Autodesk Fusion 360 part; units mm, degrees
(part 4 of 40)
  spline S18 degree 5 poles (171.8057, 195.8153) (171.7853, 195.8385) (171.7452, 195.8854) (171.6869, 195.9573) (171.6128, 196.056) (171.5254, 196.1833) (171.4416, 196.3135) (171.36, 196.4454) (171.2796, 196.5782) (171.2, 196.7117) (171.1213, 196.8458) (171.0437, 196.9807) (170.9678, 197.1168) (170.8937, 197.2543) (170.8214, 197.393) (170.7507, 197.5329) (170.6816, 197.6738) (170.6136, 197.8156) (170.5467, 197.9581) (170.4808, 198.1012) (170.416, 198.245) (170.3522, 198.3895) (170.2896, 198.5347) (170.2281, 198.6807) (170.1678, 198.8274) (170.1086, 198.9749) (170.0505, 199.123) (169.9934, 199.2717) (169.9373, 199.421) (169.8821, 199.5709) (169.8279, 199.7214) (169.7746, 199.8724) (169.7223, 200.024) (169.671, 200.1761) (169.6206, 200.3288) (169.5712, 200.482) (169.5226, 200.6358) (169.475, 200.79) (169.4283, 200.9447) (169.3825, 201.0999) (169.3375, 201.2556) (169.2934, 201.4118) (169.2502, 201.5684) (169.2079, 201.7255) (169.1664, 201.883) (169.1257, 202.0409) (169.0859, 202.1993) (169.047, 202.3581) (169.0089, 202.5173) (168.9716, 202.6769) (168.9351, 202.8369) (168.8994, 202.9973) (168.8646, 203.1581) (168.8305, 203.3193) (168.7973, 203.4809) (168.7648, 203.6428) (168.7332, 203.8051) (168.7023, 203.9677) (168.6723, 204.1307) (168.643, 204.294) (168.6145, 204.4577) (168.5867, 204.6217) (168.5597, 204.7861) (168.5336, 204.9508) (168.5081, 205.1158) (168.4834, 205.2811) (168.4595, 205.4467) (168.4364, 205.6126) (168.414, 205.7789) (168.3923, 205.9454) (168.3714, 206.1122) (168.3553, 206.2459) (168.3435, 206.3463) (168.3358, 206.4133) (168.332, 206.4469) knots 0 0 0 0 0 0 0.01428571 0.02857143 0.04285714 0.05714286 0.07142857 0.08571429 0.1 0.11428571 0.12857143 0.14285714 0.15714286 0.17142857 0.18571429 0.2 0.21428571 0.22857143 0.24285714 0.25714286 0.27142857 0.28571429 0.3 0.31428571 0.32857143 0.34285714 0.35714286 0.37142857 0.38571429 0.4 0.41428571 0.42857143 0.44285714 0.45714286 0.47142857 0.48571429 0.5 0.51428571 0.52857143 0.54285714 0.55714286 0.57142857 0.58571429 0.6 0.61428571 0.62857143 0.64285714 0.65714286 0.67142857 0.68571429 0.7 0.71428571 0.72857143 0.74285714 0.75714286 0.77142857 0.78571429 0.8 0.81428571 0.82857143 0.84285714 0.85714286 0.87142857 0.88571429 0.9 0.91428571 0.92857143 0.94285714 0.95714286 0.97142857 0.98571429 1 1 1 1 1 1
  line L1367 (171.8057, 195.8153) -> (171.7853, 195.8385) construction
  line L1368 (171.7853, 195.8385) -> (171.7452, 195.8854) construction
  line L1369 (171.7452, 195.8854) -> (171.6869, 195.9573) construction
  line L1370 (171.6869, 195.9573) -> (171.6128, 196.056) construction
  line L1371 (171.6128, 196.056) -> (171.5254, 196.1833) construction
  line L1372 (171.5254, 196.1833) -> (171.4416, 196.3135) construction
  line L1373 (171.4416, 196.3135) -> (171.36, 196.4454) construction
  line L1374 (171.36, 196.4454) -> (171.2796, 196.5782) construction
  line L1375 (171.2796, 196.5782) -> (171.2, 196.7117) construction
  line L1376 (171.2, 196.7117) -> (171.1213, 196.8458) construction
  line L1377 (171.1213, 196.8458) -> (171.0437, 196.9807) construction
  line L1378 (171.0437, 196.9807) -> (170.9678, 197.1168) construction
  line L1379 (170.9678, 197.1168) -> (170.8937, 197.2543) construction
  line L1380 (170.8937, 197.2543) -> (170.8214, 197.393) construction
  line L1381 (170.8214, 197.393) -> (170.7507, 197.5329) construction
  line L1382 (170.7507, 197.5329) -> (170.6816, 197.6738) construction
  line L1383 (170.6816, 197.6738) -> (170.6136, 197.8156) construction
  line L1384 (170.6136, 197.8156) -> (170.5467, 197.9581) construction
  line L1385 (170.5467, 197.9581) -> (170.4808, 198.1012) construction
  line L1386 (170.4808, 198.1012) -> (170.416, 198.245) construction
  line L1387 (170.416, 198.245) -> (170.3522, 198.3895) construction
  line L1388 (170.3522, 198.3895) -> (170.2896, 198.5347) construction
  line L1389 (170.2896, 198.5347) -> (170.2281, 198.6807) construction
  line L1390 (170.2281, 198.6807) -> (170.1678, 198.8274) construction
  line L1391 (170.1678, 198.8274) -> (170.1086, 198.9749) construction
  line L1392 (170.1086, 198.9749) -> (170.0505, 199.123) construction
  line L1393 (170.0505, 199.123) -> (169.9934, 199.2717) construction
  line L1394 (169.9934, 199.2717) -> (169.9373, 199.421) construction
  line L1395 (169.9373, 199.421) -> (169.8821, 199.5709) construction
  line L1396 (169.8821, 199.5709) -> (169.8279, 199.7214) construction
  line L1397 (169.8279, 199.7214) -> (169.7746, 199.8724) construction
  line L1398 (169.7746, 199.8724) -> (169.7223, 200.024) construction
  line L1399 (169.7223, 200.024) -> (169.671, 200.1761) construction
  line L1400 (169.671, 200.1761) -> (169.6206, 200.3288) construction
  line L1401 (169.6206, 200.3288) -> (169.5712, 200.482) construction
  line L1402 (169.5712, 200.482) -> (169.5226, 200.6358) construction
  line L1403 (169.5226, 200.6358) -> (169.475, 200.79) construction
  line L1404 (169.475, 200.79) -> (169.4283, 200.9447) construction
  line L1405 (169.4283, 200.9447) -> (169.3825, 201.0999) construction
  line L1406 (169.3825, 201.0999) -> (169.3375, 201.2556) construction
  line L1407 (169.3375, 201.2556) -> (169.2934, 201.4118) construction
  line L1408 (169.2934, 201.4118) -> (169.2502, 201.5684) construction
  line L1409 (169.2502, 201.5684) -> (169.2079, 201.7255) construction
  line L1410 (169.2079, 201.7255) -> (169.1664, 201.883) construction
  line L1411 (169.1664, 201.883) -> (169.1257, 202.0409) construction
  line L1412 (169.1257, 202.0409) -> (169.0859, 202.1993) construction
  line L1413 (169.0859, 202.1993) -> (169.047, 202.3581) construction
  line L1414 (169.047, 202.3581) -> (169.0089, 202.5173) construction
  line L1415 (169.0089, 202.5173) -> (168.9716, 202.6769) construction
  line L1416 (168.9716, 202.6769) -> (168.9351, 202.8369) construction
  line L1417 (168.9351, 202.8369) -> (168.8994, 202.9973) construction
  line L1418 (168.8994, 202.9973) -> (168.8646, 203.1581) construction
  line L1419 (168.8646, 203.1581) -> (168.8305, 203.3193) construction
  line L1420 (168.8305, 203.3193) -> (168.7973, 203.4809) construction
  line L1421 (168.7973, 203.4809) -> (168.7648, 203.6428) construction
  line L1422 (168.7648, 203.6428) -> (168.7332, 203.8051) construction
  line L1423 (168.7332, 203.8051) -> (168.7023, 203.9677) construction
  line L1424 (168.7023, 203.9677) -> (168.6723, 204.1307) construction
  line L1425 (168.6723, 204.1307) -> (168.643, 204.294) construction
  line L1426 (168.643, 204.294) -> (168.6145, 204.4577) construction
  line L1427 (168.6145, 204.4577) -> (168.5867, 204.6217) construction
  line L1428 (168.5867, 204.6217) -> (168.5597, 204.7861) construction
  line L1429 (168.5597, 204.7861) -> (168.5336, 204.9508) construction
  line L1430 (168.5336, 204.9508) -> (168.5081, 205.1158) construction
  line L1431 (168.5081, 205.1158) -> (168.4834, 205.2811) construction
  line L1432 (168.4834, 205.2811) -> (168.4595, 205.4467) construction
  line L1433 (168.4595, 205.4467) -> (168.4364, 205.6126) construction
  line L1434 (168.4364, 205.6126) -> (168.414, 205.7789) construction
  line L1435 (168.414, 205.7789) -> (168.3923, 205.9454) construction
  line L1436 (168.3923, 205.9454) -> (168.3714, 206.1122) construction
  line L1437 (168.3714, 206.1122) -> (168.3553, 206.2459) construction
  line L1438 (168.3553, 206.2459) -> (168.3435, 206.3463) construction
  line L1439 (168.3435, 206.3463) -> (168.3358, 206.4133) construction
  line L1440 (168.3358, 206.4133) -> (168.332, 206.4469) construction
  spline S19 degree 5 poles (171.8057, 195.8153) (171.7853, 195.8385) (171.7452, 195.8854) (171.6869, 195.9573) (171.6128, 196.056) (171.5254, 196.1833) (171.4416, 196.3135) (171.36, 196.4454) (171.2796, 196.5782) (171.2, 196.7117) (171.1213, 196.8458) (171.0437, 196.9807) (170.9678, 197.1168) (170.8937, 197.2543) (170.8214, 197.393) (170.7507, 197.5329) (170.6816, 197.6738) (170.6136, 197.8156) (170.5467, 197.9581) (170.4808, 198.1012) (170.416, 198.245) (170.3522, 198.3895) (170.2896, 198.5347) (170.2281, 198.6807) (170.1678, 198.8274) (170.1086, 198.9749) (170.0505, 199.123) (169.9934, 199.2717) (169.9373, 199.421) (169.8821, 199.5709) (169.8279, 199.7214) (169.7746, 199.8724) (169.7223, 200.024) (169.671, 200.1761) (169.6206, 200.3288) (169.5712, 200.482) (169.5226, 200.6358) (169.475, 200.79) (169.4283, 200.9447) (169.3825, 201.0999) (169.3375, 201.2556) (169.2934, 201.4118) (169.2502, 201.5684) (169.2079, 201.7255) (169.1664, 201.883) (169.1257, 202.0409) (169.0859, 202.1993) (169.047, 202.3581) (169.0089, 202.5173) (168.9716, 202.6769) (168.9351, 202.8369) (168.8994, 202.9973) (168.8646, 203.1581) (168.8305, 203.3193) (168.7973, 203.4809) (168.7648, 203.6428) (168.7332, 203.8051) (168.7023, 203.9677) (168.6723, 204.1307) (168.643, 204.294) (168.6145, 204.4577) (168.5867, 204.6217) (168.5597, 204.7861) (168.5336, 204.9508) (168.5081, 205.1158) (168.4834, 205.2811) (168.4595, 205.4467) (168.4364, 205.6126) (168.414, 205.7789) (168.3923, 205.9454) (168.3714, 206.1122) (168.3553, 206.2459) (168.3435, 206.3463) (168.3358, 206.4133) (168.332, 206.4469) knots 0 0 0 0 0 0 0.01428571 0.02857143 0.04285714 0.05714286 0.07142857 0.08571429 0.1 0.11428571 0.12857143 0.14285714 0.15714286 0.17142857 0.18571429 0.2 0.21428571 0.22857143 0.24285714 0.25714286 0.27142857 0.28571429 0.3 0.31428571 0.32857143 0.34285714 0.35714286 0.37142857 0.38571429 0.4 0.41428571 0.42857143 0.44285714 0.45714286 0.47142857 0.48571429 0.5 0.51428571 0.52857143 0.54285714 0.55714286 0.57142857 0.58571429 0.6 0.61428571 0.62857143 0.64285714 0.65714286 0.67142857 0.68571429 0.7 0.71428571 0.72857143 0.74285714 0.75714286 0.77142857 0.78571429 0.8 0.81428571 0.82857143 0.84285714 0.85714286 0.87142857 0.88571429 0.9 0.91428571 0.92857143 0.94285714 0.95714286 0.97142857 0.98571429 1 1 1 1 1 1
  line L1441 (171.8057, 195.8153) -> (171.7853, 195.8385) construction
  line L1442 (171.7853, 195.8385) -> (171.7452, 195.8854) construction
  line L1443 (171.7452, 195.8854) -> (171.6869, 195.9573) construction
  line L1444 (171.6869, 195.9573) -> (171.6128, 196.056) construction
  line L1445 (171.6128, 196.056) -> (171.5254, 196.1833) construction
  line L1446 (171.5254, 196.1833) -> (171.4416, 196.3135) construction
  line L1447 (171.4416, 196.3135) -> (171.36, 196.4454) construction
  line L1448 (171.36, 196.4454) -> (171.2796, 196.5782) construction
  line L1449 (171.2796, 196.5782) -> (171.2, 196.7117) construction
  line L1450 (171.2, 196.7117) -> (171.1213, 196.8458) construction
  line L1451 (171.1213, 196.8458) -> (171.0437, 196.9807) construction
  line L1452 (171.0437, 196.9807) -> (170.9678, 197.1168) construction
  line L1453 (170.9678, 197.1168) -> (170.8937, 197.2543) construction
  line L1454 (170.8937, 197.2543) -> (170.8214, 197.393) construction
  line L1455 (170.8214, 197.393) -> (170.7507, 197.5329) construction
  line L1456 (170.7507, 197.5329) -> (170.6816, 197.6738) construction
  line L1457 (170.6816, 197.6738) -> (170.6136, 197.8156) construction
  line L1458 (170.6136, 197.8156) -> (170.5467, 197.9581) construction
  line L1459 (170.5467, 197.9581) -> (170.4808, 198.1012) construction
  line L1460 (170.4808, 198.1012) -> (170.416, 198.245) construction
  line L1461 (170.416, 198.245) -> (170.3522, 198.3895) construction
  line L1462 (170.3522, 198.3895) -> (170.2896, 198.5347) construction
  line L1463 (170.2896, 198.5347) -> (170.2281, 198.6807) construction
  line L1464 (170.2281, 198.6807) -> (170.1678, 198.8274) construction
  line L1465 (170.1678, 198.8274) -> (170.1086, 198.9749) construction
  line L1466 (170.1086, 198.9749) -> (170.0505, 199.123) construction
  line L1467 (170.0505, 199.123) -> (169.9934, 199.2717) construction
  line L1468 (169.9934, 199.2717) -> (169.9373, 199.421) construction
  line L1469 (169.9373, 199.421) -> (169.8821, 199.5709) construction
  line L1470 (169.8821, 199.5709) -> (169.8279, 199.7214) construction
  line L1471 (169.8279, 199.7214) -> (169.7746, 199.8724) construction
  line L1472 (169.7746, 199.8724) -> (169.7223, 200.024) construction
  line L1473 (169.7223, 200.024) -> (169.671, 200.1761) construction
  line L1474 (169.671, 200.1761) -> (169.6206, 200.3288) construction
  line L1475 (169.6206, 200.3288) -> (169.5712, 200.482) construction
  line L1476 (169.5712, 200.482) -> (169.5226, 200.6358) construction
  line L1477 (169.5226, 200.6358) -> (169.475, 200.79) construction
  line L1478 (169.475, 200.79) -> (169.4283, 200.9447) construction
  line L1479 (169.4283, 200.9447) -> (169.3825, 201.0999) construction
  line L1480 (169.3825, 201.0999) -> (169.3375, 201.2556) construction
  line L1481 (169.3375, 201.2556) -> (169.2934, 201.4118) construction
  line L1482 (169.2934, 201.4118) -> (169.2502, 201.5684) construction
  line L1483 (169.2502, 201.5684) -> (169.2079, 201.7255) construction
  line L1484 (169.2079, 201.7255) -> (169.1664, 201.883) construction
  line L1485 (169.1664, 201.883) -> (169.1257, 202.0409) construction
  line L1486 (169.1257, 202.0409) -> (169.0859, 202.1993) construction
  line L1487 (169.0859, 202.1993) -> (169.047, 202.3581) construction
  line L1488 (169.047, 202.3581) -> (169.0089, 202.5173) construction
  line L1489 (169.0089, 202.5173) -> (168.9716, 202.6769) construction
  line L1490 (168.9716, 202.6769) -> (168.9351, 202.8369) construction
  line L1491 (168.9351, 202.8369) -> (168.8994, 202.9973) construction
  line L1492 (168.8994, 202.9973) -> (168.8646, 203.1581) construction
  line L1493 (168.8646, 203.1581) -> (168.8305, 203.3193) construction
  line L1494 (168.8305, 203.3193) -> (168.7973, 203.4809) construction
  line L1495 (168.7973, 203.4809) -> (168.7648, 203.6428) construction
  line L1496 (168.7648, 203.6428) -> (168.7332, 203.8051) construction
  line L1497 (168.7332, 203.8051) -> (168.7023, 203.9677) construction
  line L1498 (168.7023, 203.9677) -> (168.6723, 204.1307) construction
  line L1499 (168.6723, 204.1307) -> (168.643, 204.294) construction
  line L1500 (168.643, 204.294) -> (168.6145, 204.4577) construction
  line L1501 (168.6145, 204.4577) -> (168.5867, 204.6217) construction
  line L1502 (168.5867, 204.6217) -> (168.5597, 204.7861) construction
  line L1503 (168.5597, 204.7861) -> (168.5336, 204.9508) construction
  line L1504 (168.5336, 204.9508) -> (168.5081, 205.1158) construction
  line L1505 (168.5081, 205.1158) -> (168.4834, 205.2811) construction
  line L1506 (168.4834, 205.2811) -> (168.4595, 205.4467) construction
  line L1507 (168.4595, 205.4467) -> (168.4364, 205.6126) construction
  line L1508 (168.4364, 205.6126) -> (168.414, 205.7789) construction
  line L1509 (168.414, 205.7789) -> (168.3923, 205.9454) construction
  line L1510 (168.3923, 205.9454) -> (168.3714, 206.1122) construction
  line L1511 (168.3714, 206.1122) -> (168.3553, 206.2459) construction
  line L1512 (168.3553, 206.2459) -> (168.3435, 206.3463) construction
  line L1513 (168.3435, 206.3463) -> (168.3358, 206.4133) construction
  line L1514 (168.3358, 206.4133) -> (168.332, 206.4469) construction
  arc A49 (242.4118, 98.8934) -> (239.7302, 99.6279) centre (240.6912, 97.8739) ccw
  arc A50 (242.4118, 98.8934) -> (239.7302, 99.6279) centre (240.6912, 97.8739) ccw
  line L1515 (251.3803, 105.4094) -> (252.4583, 104.1847)
  line L1516 (251.3803, 105.4094) -> (252.4583, 104.1847)
  line L1517 (242.4118, 98.8934) -> (243.2435, 97.4897)
  line L1518 (242.4118, 98.8934) -> (243.2435, 97.4897)
  arc A51 (236.6621, 98.0646) -> (239.7302, 99.6279) centre (212.132, 150) ccw
  arc A52 (251.5104, 108.1868) -> (251.3803, 105.4094) centre (252.8816, 106.7308) ccw
  arc A53 (264.0674, 174.5301) -> (262.5041, 177.5982) centre (212.132, 150) ccw
  arc A54 (236.6621, 98.0646) -> (239.7302, 99.6279) centre (212.132, 150) ccw
  arc A55 (264.0674, 174.5301) -> (266.6686, 173.5481) centre (265.8758, 175.3842) ccw
  arc A56 (251.5104, 108.1868) -> (251.3803, 105.4094) centre (252.8816, 106.7308) ccw
  spline S20 degree 5 poles (272.9005, 144.3049) (272.9313, 144.3021) (272.9929, 144.2971) (273.0853, 144.2922) (273.2086, 144.2903) (273.363, 144.2944) (273.5176, 144.3031) (273.6723, 144.3146) (273.827, 144.3277) (273.9818, 144.3417) (274.1365, 144.3569) (274.2913, 144.3735) (274.446, 144.392) (274.6008, 144.4129) (274.7555, 144.4359) (274.9102, 144.461) (275.0649, 144.4879) (275.2195, 144.5162) (275.3741, 144.5458) (275.5286, 144.5767) (275.6831, 144.6087) (275.8375, 144.6421) (275.9918, 144.6768) (276.146, 144.7129) (276.3002, 144.7503) (276.4542, 144.7891) (276.6082, 144.8291) (276.7621, 144.8703) (276.9159, 144.9127) (277.0696, 144.9561) (277.2232, 145.0007) (277.3767, 145.0464) (277.53, 145.0932) (277.6833, 145.1411) (277.8364, 145.1901) (277.9894, 145.2401) (278.1423, 145.2913) (278.2951, 145.3434) (278.4478, 145.3965) (278.6003, 145.4507) (278.7526, 145.5058) (278.9049, 145.562) (279.057, 145.619) (279.209, 145.6771) (279.3608, 145.7361) (279.5124, 145.7961) (279.664, 145.857) (279.8153, 145.9188) (279.9665, 145.9815) (280.1176, 146.0452) (280.2685, 146.1097) (280.4192, 146.1751) (280.5698, 146.2415) (280.7202, 146.3087) (280.8704, 146.3767) (281.0205, 146.4457) (281.1704, 146.5154) (281.3201, 146.5861) (281.4696, 146.6575) (281.619, 146.7299) (281.7682, 146.803) (281.9172, 146.877) (282.066, 146.9518) (282.2146, 147.0274) (282.3631, 147.1038) (282.5113, 147.181) (282.6594, 147.259) (282.8072, 147.3378) (282.9549, 147.4174) (283.1023, 147.4977) (283.2496, 147.5789) (283.3672, 147.6444) (283.4554, 147.6939) (283.5141, 147.7271) (283.5435, 147.7437) knots 0 0 0 0 0 0 0.01428571 0.02857143 0.04285714 0.05714286 0.07142857 0.08571429 0.1 0.11428571 0.12857143 0.14285714 0.15714286 0.17142857 0.18571429 0.2 0.21428571 0.22857143 0.24285714 0.25714286 0.27142857 0.28571429 0.3 0.31428571 0.32857143 0.34285714 0.35714286 0.37142857 0.38571429 0.4 0.41428571 0.42857143 0.44285714 0.45714286 0.47142857 0.48571429 0.5 0.51428571 0.52857143 0.54285714 0.55714286 0.57142857 0.58571429 0.6 0.61428571 0.62857143 0.64285714 0.65714286 0.67142857 0.68571429 0.7 0.71428571 0.72857143 0.74285714 0.75714286 0.77142857 0.78571429 0.8 0.81428571 0.82857143 0.84285714 0.85714286 0.87142857 0.88571429 0.9 0.91428571 0.92857143 0.94285714 0.95714286 0.97142857 0.98571429 1 1 1 1 1 1
  line L1519 (272.9005, 144.3049) -> (272.9313, 144.3021) construction
  line L1520 (272.9313, 144.3021) -> (272.9929, 144.2971) construction
  line L1521 (272.9929, 144.2971) -> (273.0853, 144.2922) construction
  line L1522 (273.0853, 144.2922) -> (273.2086, 144.2903) construction
  line L1523 (273.2086, 144.2903) -> (273.363, 144.2944) construction
  line L1524 (273.363, 144.2944) -> (273.5176, 144.3031) construction
  line L1525 (273.5176, 144.3031) -> (273.6723, 144.3146) construction
  line L1526 (273.6723, 144.3146) -> (273.827, 144.3277) construction
  line L1527 (273.827, 144.3277) -> (273.9818, 144.3417) construction
  line L1528 (273.9818, 144.3417) -> (274.1365, 144.3569) construction
  line L1529 (274.1365, 144.3569) -> (274.2913, 144.3735) construction
  line L1530 (274.2913, 144.3735) -> (274.446, 144.392) construction
  line L1531 (274.446, 144.392) -> (274.6008, 144.4129) construction
  line L1532 (274.6008, 144.4129) -> (274.7555, 144.4359) construction
  line L1533 (274.7555, 144.4359) -> (274.9102, 144.461) construction
  line L1534 (274.9102, 144.461) -> (275.0649, 144.4879) construction
  line L1535 (275.0649, 144.4879) -> (275.2195, 144.5162) construction
  line L1536 (275.2195, 144.5162) -> (275.3741, 144.5458) construction
  line L1537 (275.3741, 144.5458) -> (275.5286, 144.5767) construction
  line L1538 (275.5286, 144.5767) -> (275.6831, 144.6087) construction
  line L1539 (275.6831, 144.6087) -> (275.8375, 144.6421) construction
  line L1540 (275.8375, 144.6421) -> (275.9918, 144.6768) construction
  line L1541 (275.9918, 144.6768) -> (276.146, 144.7129) construction
  line L1542 (276.146, 144.7129) -> (276.3002, 144.7503) construction
  line L1543 (276.3002, 144.7503) -> (276.4542, 144.7891) construction
  line L1544 (276.4542, 144.7891) -> (276.6082, 144.8291) construction
  line L1545 (276.6082, 144.8291) -> (276.7621, 144.8703) construction
  line L1546 (276.7621, 144.8703) -> (276.9159, 144.9127) construction
  line L1547 (276.9159, 144.9127) -> (277.0696, 144.9561) construction
  line L1548 (277.0696, 144.9561) -> (277.2232, 145.0007) construction
  line L1549 (277.2232, 145.0007) -> (277.3767, 145.0464) construction
  line L1550 (277.3767, 145.0464) -> (277.53, 145.0932) construction
  line L1551 (277.53, 145.0932) -> (277.6833, 145.1411) construction
  line L1552 (277.6833, 145.1411) -> (277.8364, 145.1901) construction
  line L1553 (277.8364, 145.1901) -> (277.9894, 145.2401) construction
  line L1554 (277.9894, 145.2401) -> (278.1423, 145.2913) construction
  line L1555 (278.1423, 145.2913) -> (278.2951, 145.3434) construction
  line L1556 (278.2951, 145.3434) -> (278.4478, 145.3965) construction
  line L1557 (278.4478, 145.3965) -> (278.6003, 145.4507) construction
  line L1558 (278.6003, 145.4507) -> (278.7526, 145.5058) construction
  line L1559 (278.7526, 145.5058) -> (278.9049, 145.562) construction
  line L1560 (278.9049, 145.562) -> (279.057, 145.619) construction
  line L1561 (279.057, 145.619) -> (279.209, 145.6771) construction
  line L1562 (279.209, 145.6771) -> (279.3608, 145.7361) construction
  line L1563 (279.3608, 145.7361) -> (279.5124, 145.7961) construction
  line L1564 (279.5124, 145.7961) -> (279.664, 145.857) construction
  line L1565 (279.664, 145.857) -> (279.8153, 145.9188) construction
  line L1566 (279.8153, 145.9188) -> (279.9665, 145.9815) construction
  line L1567 (279.9665, 145.9815) -> (280.1176, 146.0452) construction
  line L1568 (280.1176, 146.0452) -> (280.2685, 146.1097) construction
  line L1569 (280.2685, 146.1097) -> (280.4192, 146.1751) construction
  line L1570 (280.4192, 146.1751) -> (280.5698, 146.2415) construction
  line L1571 (280.5698, 146.2415) -> (280.7202, 146.3087) construction
  line L1572 (280.7202, 146.3087) -> (280.8704, 146.3767) construction
  line L1573 (280.8704, 146.3767) -> (281.0205, 146.4457) construction
  line L1574 (281.0205, 146.4457) -> (281.1704, 146.5154) construction
  line L1575 (281.1704, 146.5154) -> (281.3201, 146.5861) construction
  line L1576 (281.3201, 146.5861) -> (281.4696, 146.6575) construction
  line L1577 (281.4696, 146.6575) -> (281.619, 146.7299) construction
  line L1578 (281.619, 146.7299) -> (281.7682, 146.803) construction
  line L1579 (281.7682, 146.803) -> (281.9172, 146.877) construction
  line L1580 (281.9172, 146.877) -> (282.066, 146.9518) construction
  line L1581 (282.066, 146.9518) -> (282.2146, 147.0274) construction
  line L1582 (282.2146, 147.0274) -> (282.3631, 147.1038) construction
  line L1583 (282.3631, 147.1038) -> (282.5113, 147.181) construction
  line L1584 (282.5113, 147.181) -> (282.6594, 147.259) construction
  line L1585 (282.6594, 147.259) -> (282.8072, 147.3378) construction
  line L1586 (282.8072, 147.3378) -> (282.9549, 147.4174) construction
  line L1587 (282.9549, 147.4174) -> (283.1023, 147.4977) construction
  line L1588 (283.1023, 147.4977) -> (283.2496, 147.5789) construction
  line L1589 (283.2496, 147.5789) -> (283.3672, 147.6444) construction
  line L1590 (283.3672, 147.6444) -> (283.4554, 147.6939) construction
  line L1591 (283.4554, 147.6939) -> (283.5141, 147.7271) construction
  line L1592 (283.5141, 147.7271) -> (283.5435, 147.7437) construction
  spline S21 degree 5 poles (272.9005, 144.3049) (272.9313, 144.3021) (272.9929, 144.2971) (273.0853, 144.2922) (273.2086, 144.2903) (273.363, 144.2944) (273.5176, 144.3031) (273.6723, 144.3146) (273.827, 144.3277) (273.9818, 144.3417) (274.1365, 144.3569) (274.2913, 144.3735) (274.446, 144.392) (274.6008, 144.4129) (274.7555, 144.4359) (274.9102, 144.461) (275.0649, 144.4879) (275.2195, 144.5162) (275.3741, 144.5458) (275.5286, 144.5767) (275.6831, 144.6087) (275.8375, 144.6421) (275.9918, 144.6768) (276.146, 144.7129) (276.3002, 144.7503) (276.4542, 144.7891) (276.6082, 144.8291) (276.7621, 144.8703) (276.9159, 144.9127) (277.0696, 144.9561) (277.2232, 145.0007) (277.3767, 145.0464) (277.53, 145.0932) (277.6833, 145.1411) (277.8364, 145.1901) (277.9894, 145.2401) (278.1423, 145.2913) (278.2951, 145.3434) (278.4478, 145.3965) (278.6003, 145.4507) (278.7526, 145.5058) (278.9049, 145.562) (279.057, 145.619) (279.209, 145.6771) (279.3608, 145.7361) (279.5124, 145.7961) (279.664, 145.857) (279.8153, 145.9188) (279.9665, 145.9815) (280.1176, 146.0452) (280.2685, 146.1097) (280.4192, 146.1751) (280.5698, 146.2415) (280.7202, 146.3087) (280.8704, 146.3767) (281.0205, 146.4457) (281.1704, 146.5154) (281.3201, 146.5861) (281.4696, 146.6575) (281.619, 146.7299) (281.7682, 146.803) (281.9172, 146.877) (282.066, 146.9518) (282.2146, 147.0274) (282.3631, 147.1038) (282.5113, 147.181) (282.6594, 147.259) (282.8072, 147.3378) (282.9549, 147.4174) (283.1023, 147.4977) (283.2496, 147.5789) (283.3672, 147.6444) (283.4554, 147.6939) (283.5141, 147.7271) (283.5435, 147.7437) knots 0 0 0 0 0 0 0.01428571 0.02857143 0.04285714 0.05714286 0.07142857 0.08571429 0.1 0.11428571 0.12857143 0.14285714 0.15714286 0.17142857 0.18571429 0.2 0.21428571 0.22857143 0.24285714 0.25714286 0.27142857 0.28571429 0.3 0.31428571 0.32857143 0.34285714 0.35714286 0.37142857 0.38571429 0.4 0.41428571 0.42857143 0.44285714 0.45714286 0.47142857 0.48571429 0.5 0.51428571 0.52857143 0.54285714 0.55714286 0.57142857 0.58571429 0.6 0.61428571 0.62857143 0.64285714 0.65714286 0.67142857 0.68571429 0.7 0.71428571 0.72857143 0.74285714 0.75714286 0.77142857 0.78571429 0.8 0.81428571 0.82857143 0.84285714 0.85714286 0.87142857 0.88571429 0.9 0.91428571 0.92857143 0.94285714 0.95714286 0.97142857 0.98571429 1 1 1 1 1 1
  line L1593 (272.9005, 144.3049) -> (272.9313, 144.3021) construction
  line L1594 (272.9313, 144.3021) -> (272.9929, 144.2971) construction
  line L1595 (272.9929, 144.2971) -> (273.0853, 144.2922) construction
  line L1596 (273.0853, 144.2922) -> (273.2086, 144.2903) construction
  line L1597 (273.2086, 144.2903) -> (273.363, 144.2944) construction
  line L1598 (273.363, 144.2944) -> (273.5176, 144.3031) construction
  line L1599 (273.5176, 144.3031) -> (273.6723, 144.3146) construction
  line L1600 (273.6723, 144.3146) -> (273.827, 144.3277) construction
  line L1601 (273.827, 144.3277) -> (273.9818, 144.3417) construction
  line L1602 (273.9818, 144.3417) -> (274.1365, 144.3569) construction
  line L1603 (274.1365, 144.3569) -> (274.2913, 144.3735) construction
  line L1604 (274.2913, 144.3735) -> (274.446, 144.392) construction
  line L1605 (274.446, 144.392) -> (274.6008, 144.4129) construction
  line L1606 (274.6008, 144.4129) -> (274.7555, 144.4359) construction
  line L1607 (274.7555, 144.4359) -> (274.9102, 144.461) construction
  line L1608 (274.9102, 144.461) -> (275.0649, 144.4879) construction
  line L1609 (275.0649, 144.4879) -> (275.2195, 144.5162) construction
  line L1610 (275.2195, 144.5162) -> (275.3741, 144.5458) construction
  line L1611 (275.3741, 144.5458) -> (275.5286, 144.5767) construction
  line L1612 (275.5286, 144.5767) -> (275.6831, 144.6087) construction
  line L1613 (275.6831, 144.6087) -> (275.8375, 144.6421) construction
  line L1614 (275.8375, 144.6421) -> (275.9918, 144.6768) construction
  line L1615 (275.9918, 144.6768) -> (276.146, 144.7129) construction
  line L1616 (276.146, 144.7129) -> (276.3002, 144.7503) construction
  line L1617 (276.3002, 144.7503) -> (276.4542, 144.7891) construction
  line L1618 (276.4542, 144.7891) -> (276.6082, 144.8291) construction
  line L1619 (276.6082, 144.8291) -> (276.7621, 144.8703) construction
  line L1620 (276.7621, 144.8703) -> (276.9159, 144.9127) construction
  line L1621 (276.9159, 144.9127) -> (277.0696, 144.9561) construction
  line L1622 (277.0696, 144.9561) -> (277.2232, 145.0007) construction
  line L1623 (277.2232, 145.0007) -> (277.3767, 145.0464) construction
  line L1624 (277.3767, 145.0464) -> (277.53, 145.0932) construction
  line L1625 (277.53, 145.0932) -> (277.6833, 145.1411) construction
  line L1626 (277.6833, 145.1411) -> (277.8364, 145.1901) construction
  line L1627 (277.8364, 145.1901) -> (277.9894, 145.2401) construction
  line L1628 (277.9894, 145.2401) -> (278.1423, 145.2913) construction
  line L1629 (278.1423, 145.2913) -> (278.2951, 145.3434) construction
  line L1630 (278.2951, 145.3434) -> (278.4478, 145.3965) construction
  line L1631 (278.4478, 145.3965) -> (278.6003, 145.4507) construction
  line L1632 (278.6003, 145.4507) -> (278.7526, 145.5058) construction
  line L1633 (278.7526, 145.5058) -> (278.9049, 145.562) construction
  line L1634 (278.9049, 145.562) -> (279.057, 145.619) construction
  line L1635 (279.057, 145.619) -> (279.209, 145.6771) construction
  line L1636 (279.209, 145.6771) -> (279.3608, 145.7361) construction
  line L1637 (279.3608, 145.7361) -> (279.5124, 145.7961) construction
  line L1638 (279.5124, 145.7961) -> (279.664, 145.857) construction
  line L1639 (279.664, 145.857) -> (279.8153, 145.9188) construction
  line L1640 (279.8153, 145.9188) -> (279.9665, 145.9815) construction
  line L1641 (279.9665, 145.9815) -> (280.1176, 146.0452) construction
  line L1642 (280.1176, 146.0452) -> (280.2685, 146.1097) construction
  line L1643 (280.2685, 146.1097) -> (280.4192, 146.1751) construction
  line L1644 (280.4192, 146.1751) -> (280.5698, 146.2415) construction
  line L1645 (280.5698, 146.2415) -> (280.7202, 146.3087) construction
  line L1646 (280.7202, 146.3087) -> (280.8704, 146.3767) construction
  line L1647 (280.8704, 146.3767) -> (281.0205, 146.4457) construction
  line L1648 (281.0205, 146.4457) -> (281.1704, 146.5154) construction
  line L1649 (281.1704, 146.5154) -> (281.3201, 146.5861) construction
  line L1650 (281.3201, 146.5861) -> (281.4696, 146.6575) construction
  line L1651 (281.4696, 146.6575) -> (281.619, 146.7299) construction
  line L1652 (281.619, 146.7299) -> (281.7682, 146.803) construction
  line L1653 (281.7682, 146.803) -> (281.9172, 146.877) construction
  line L1654 (281.9172, 146.877) -> (282.066, 146.9518) construction
  line L1655 (282.066, 146.9518) -> (282.2146, 147.0274) construction
  line L1656 (282.2146, 147.0274) -> (282.3631, 147.1038) construction
  line L1657 (282.3631, 147.1038) -> (282.5113, 147.181) construction
  line L1658 (282.5113, 147.181) -> (282.6594, 147.259) construction
  line L1659 (282.6594, 147.259) -> (282.8072, 147.3378) construction
  line L1660 (282.8072, 147.3378) -> (282.9549, 147.4174) construction
  line L1661 (282.9549, 147.4174) -> (283.1023, 147.4977) construction
  line L1662 (283.1023, 147.4977) -> (283.2496, 147.5789) construction
  line L1663 (283.2496, 147.5789) -> (283.3672, 147.6444) construction
  line L1664 (283.3672, 147.6444) -> (283.4554, 147.6939) construction
  line L1665 (283.4554, 147.6939) -> (283.5141, 147.7271) construction
  line L1666 (283.5141, 147.7271) -> (283.5435, 147.7437) construction
  arc A57 (219.4126, 93.0263) -> (222.8136, 93.565) centre (212.132, 150) ccw
  arc A58 (219.4126, 93.0263) -> (222.8136, 93.565) centre (212.132, 150) ccw
  line L1667 (266.6686, 173.5481) -> (268.1665, 174.1948)
  arc A59 (225.137, 92.0377) -> (222.8136, 93.565) centre (223.1855, 91.5999) ccw
  arc A60 (225.137, 92.0377) -> (222.8136, 93.565) centre (223.1855, 91.5999) ccw
  spline S22 degree 5 poles (225.4942, 90.4458) (225.501, 90.4157) (225.5153, 90.3556) (225.5391, 90.2662) (225.5755, 90.1483) (225.6271, 90.0027) (225.6831, 89.8584) (225.7419, 89.7148) (225.8021, 89.5717) (225.8633, 89.4289) (225.9255, 89.2864) (225.9891, 89.1443) (226.0546, 89.0029) (226.1222, 88.8621) (226.192, 88.7221) (226.2636, 88.5827) (226.337, 88.4439) (226.4117, 88.3056) (226.4877, 88.1678) (226.5647, 88.0303) (226.6429, 87.8933) (226.7224, 87.7568) (226.8031, 87.6208) (226.885, 87.4852) (226.9683, 87.3502) (227.0528, 87.2157) (227.1384, 87.0816) (227.2252, 86.948) (227.313, 86.8148) (227.4018, 86.682) (227.4917, 86.5497) (227.5826, 86.4179) (227.6745, 86.2865) (227.7674, 86.1555) (227.8613, 86.025) (227.9562, 85.895) (228.052, 85.7654) (228.1488, 85.6362) (228.2466, 85.5074) (228.3452, 85.3791) (228.4447, 85.2512) (228.5451, 85.1238) (228.6464, 84.9968) (228.7486, 84.8702) (228.8516, 84.744) (228.9555, 84.6183) (229.0603, 84.493) (229.1658, 84.3682) (229.2722, 84.2438) (229.3794, 84.1198) (229.4875, 83.9962) (229.5963, 83.8731) (229.7059, 83.7503) (229.8162, 83.6281) (229.9274, 83.5062) (230.0393, 83.3848) (230.152, 83.2638) (230.2655, 83.1432) (230.3797, 83.0231) (230.4946, 82.9034) (230.6102, 82.7841) (230.7266, 82.6653) (230.8438, 82.5469) (230.9616, 82.4289) (231.0801, 82.3113) (231.1994, 82.1942) (231.3193, 82.0775) (231.4399, 81.9612) (231.5613, 81.8454) (231.6832, 81.73) (231.8059, 81.615) (231.9046, 81.5233) (231.9789, 81.4548) (232.0286, 81.4092) (232.0535, 81.3864) knots 0 0 0 0 0 0 0.01428571 0.02857143 0.04285714 0.05714286 0.07142857 0.08571429 0.1 0.11428571 0.12857143 0.14285714 0.15714286 0.17142857 0.18571429 0.2 0.21428571 0.22857143 0.24285714 0.25714286 0.27142857 0.28571429 0.3 0.31428571 0.32857143 0.34285714 0.35714286 0.37142857 0.38571429 0.4 0.41428571 0.42857143 0.44285714 0.45714286 0.47142857 0.48571429 0.5 0.51428571 0.52857143 0.54285714 0.55714286 0.57142857 0.58571429 0.6 0.61428571 0.62857143 0.64285714 0.65714286 0.67142857 0.68571429 0.7 0.71428571 0.72857143 0.74285714 0.75714286 0.77142857 0.78571429 0.8 0.81428571 0.82857143 0.84285714 0.85714286 0.87142857 0.88571429 0.9 0.91428571 0.92857143 0.94285714 0.95714286 0.97142857 0.98571429 1 1 1 1 1 1
  line L1668 (225.4942, 90.4458) -> (225.501, 90.4157) construction
  line L1669 (225.501, 90.4157) -> (225.5153, 90.3556) construction
  line L1670 (225.5153, 90.3556) -> (225.5391, 90.2662) construction
  line L1671 (225.5391, 90.2662) -> (225.5755, 90.1483) construction
  line L1672 (225.5755, 90.1483) -> (225.6271, 90.0027) construction
  line L1673 (225.6271, 90.0027) -> (225.6831, 89.8584) construction
  line L1674 (225.6831, 89.8584) -> (225.7419, 89.7148) construction
  line L1675 (225.7419, 89.7148) -> (225.8021, 89.5717) construction
  line L1676 (225.8021, 89.5717) -> (225.8633, 89.4289) construction
  line L1677 (225.8633, 89.4289) -> (225.9255, 89.2864) construction
  line L1678 (225.9255, 89.2864) -> (225.9891, 89.1443) construction
  line L1679 (225.9891, 89.1443) -> (226.0546, 89.0029) construction
  line L1680 (226.0546, 89.0029) -> (226.1222, 88.8621) construction
  line L1681 (226.1222, 88.8621) -> (226.192, 88.7221) construction
  line L1682 (226.192, 88.7221) -> (226.2636, 88.5827) construction
  line L1683 (226.2636, 88.5827) -> (226.337, 88.4439) construction
  line L1684 (226.337, 88.4439) -> (226.4117, 88.3056) construction
  line L1685 (226.4117, 88.3056) -> (226.4877, 88.1678) construction
  line L1686 (226.4877, 88.1678) -> (226.5647, 88.0303) construction
  line L1687 (226.5647, 88.0303) -> (226.6429, 87.8933) construction
  line L1688 (226.6429, 87.8933) -> (226.7224, 87.7568) construction
  line L1689 (226.7224, 87.7568) -> (226.8031, 87.6208) construction
  line L1690 (226.8031, 87.6208) -> (226.885, 87.4852) construction
  line L1691 (226.885, 87.4852) -> (226.9683, 87.3502) construction
  line L1692 (226.9683, 87.3502) -> (227.0528, 87.2157) construction
  line L1693 (227.0528, 87.2157) -> (227.1384, 87.0816) construction
  line L1694 (227.1384, 87.0816) -> (227.2252, 86.948) construction
  line L1695 (227.2252, 86.948) -> (227.313, 86.8148) construction
  line L1696 (227.313, 86.8148) -> (227.4018, 86.682) construction
  line L1697 (227.4018, 86.682) -> (227.4917, 86.5497) construction
  line L1698 (227.4917, 86.5497) -> (227.5826, 86.4179) construction
  line L1699 (227.5826, 86.4179) -> (227.6745, 86.2865) construction
  line L1700 (227.6745, 86.2865) -> (227.7674, 86.1555) construction
  line L1701 (227.7674, 86.1555) -> (227.8613, 86.025) construction
  line L1702 (227.8613, 86.025) -> (227.9562, 85.895) construction
  line L1703 (227.9562, 85.895) -> (228.052, 85.7654) construction
  line L1704 (228.052, 85.7654) -> (228.1488, 85.6362) construction
  line L1705 (228.1488, 85.6362) -> (228.2466, 85.5074) construction
  line L1706 (228.2466, 85.5074) -> (228.3452, 85.3791) construction
  line L1707 (228.3452, 85.3791) -> (228.4447, 85.2512) construction
  line L1708 (228.4447, 85.2512) -> (228.5451, 85.1238) construction
  line L1709 (228.5451, 85.1238) -> (228.6464, 84.9968) construction
  line L1710 (228.6464, 84.9968) -> (228.7486, 84.8702) construction
  line L1711 (228.7486, 84.8702) -> (228.8516, 84.744) construction
  line L1712 (228.8516, 84.744) -> (228.9555, 84.6183) construction
  line L1713 (228.9555, 84.6183) -> (229.0603, 84.493) construction
  line L1714 (229.0603, 84.493) -> (229.1658, 84.3682) construction
  line L1715 (229.1658, 84.3682) -> (229.2722, 84.2438) construction
  line L1716 (229.2722, 84.2438) -> (229.3794, 84.1198) construction
  line L1717 (229.3794, 84.1198) -> (229.4875, 83.9962) construction
  line L1718 (229.4875, 83.9962) -> (229.5963, 83.8731) construction
  line L1719 (229.5963, 83.8731) -> (229.7059, 83.7503) construction
  line L1720 (229.7059, 83.7503) -> (229.8162, 83.6281) construction
  line L1721 (229.8162, 83.6281) -> (229.9274, 83.5062) construction
  line L1722 (229.9274, 83.5062) -> (230.0393, 83.3848) construction
  line L1723 (230.0393, 83.3848) -> (230.152, 83.2638) construction
  line L1724 (230.152, 83.2638) -> (230.2655, 83.1432) construction
  line L1725 (230.2655, 83.1432) -> (230.3797, 83.0231) construction
  line L1726 (230.3797, 83.0231) -> (230.4946, 82.9034) construction
  line L1727 (230.4946, 82.9034) -> (230.6102, 82.7841) construction
  line L1728 (230.6102, 82.7841) -> (230.7266, 82.6653) construction
  line L1729 (230.7266, 82.6653) -> (230.8438, 82.5469) construction
  line L1730 (230.8438, 82.5469) -> (230.9616, 82.4289) construction
  line L1731 (230.9616, 82.4289) -> (231.0801, 82.3113) construction
  line L1732 (231.0801, 82.3113) -> (231.1994, 82.1942) construction
  line L1733 (231.1994, 82.1942) -> (231.3193, 82.0775) construction
  line L1734 (231.3193, 82.0775) -> (231.4399, 81.9612) construction
  line L1735 (231.4399, 81.9612) -> (231.5613, 81.8454) construction
  line L1736 (231.5613, 81.8454) -> (231.6832, 81.73) construction
  line L1737 (231.6832, 81.73) -> (231.8059, 81.615) construction
  line L1738 (231.8059, 81.615) -> (231.9046, 81.5233) construction
  line L1739 (231.9046, 81.5233) -> (231.9789, 81.4548) construction
  line L1740 (231.9789, 81.4548) -> (232.0286, 81.4092) construction
  line L1741 (232.0286, 81.4092) -> (232.0535, 81.3864) construction
  spline S23 degree 5 poles (225.4942, 90.4458) (225.501, 90.4157) (225.5153, 90.3556) (225.5391, 90.2662) (225.5755, 90.1483) (225.6271, 90.0027) (225.6831, 89.8584) (225.7419, 89.7148) (225.8021, 89.5717) (225.8633, 89.4289) (225.9255, 89.2864) (225.9891, 89.1443) (226.0546, 89.0029) (226.1222, 88.8621) (226.192, 88.7221) (226.2636, 88.5827) (226.337, 88.4439) (226.4117, 88.3056) (226.4877, 88.1678) (226.5647, 88.0303) (226.6429, 87.8933) (226.7224, 87.7568) (226.8031, 87.6208) (226.885, 87.4852) (226.9683, 87.3502) (227.0528, 87.2157) (227.1384, 87.0816) (227.2252, 86.948) (227.313, 86.8148) (227.4018, 86.682) (227.4917, 86.5497) (227.5826, 86.4179) (227.6745, 86.2865) (227.7674, 86.1555) (227.8613, 86.025) (227.9562, 85.895) (228.052, 85.7654) (228.1488, 85.6362) (228.2466, 85.5074) (228.3452, 85.3791) (228.4447, 85.2512) (228.5451, 85.1238) (228.6464, 84.9968) (228.7486, 84.8702) (228.8516, 84.744) (228.9555, 84.6183) (229.0603, 84.493) (229.1658, 84.3682) (229.2722, 84.2438) (229.3794, 84.1198) (229.4875, 83.9962) (229.5963, 83.8731) (229.7059, 83.7503) (229.8162, 83.6281) (229.9274, 83.5062) (230.0393, 83.3848) (230.152, 83.2638) (230.2655, 83.1432) (230.3797, 83.0231) (230.4946, 82.9034) (230.6102, 82.7841) (230.7266, 82.6653) (230.8438, 82.5469) (230.9616, 82.4289) (231.0801, 82.3113) (231.1994, 82.1942) (231.3193, 82.0775) (231.4399, 81.9612) (231.5613, 81.8454) (231.6832, 81.73) (231.8059, 81.615) (231.9046, 81.5233) (231.9789, 81.4548) (232.0286, 81.4092) (232.0535, 81.3864) knots 0 0 0 0 0 0 0.01428571 0.02857143 0.04285714 0.05714286 0.07142857 0.08571429 0.1 0.11428571 0.12857143 0.14285714 0.15714286 0.17142857 0.18571429 0.2 0.21428571 0.22857143 0.24285714 0.25714286 0.27142857 0.28571429 0.3 0.31428571 0.32857143 0.34285714 0.35714286 0.37142857 0.38571429 0.4 0.41428571 0.42857143 0.44285714 0.45714286 0.47142857 0.48571429 0.5 0.51428571 0.52857143 0.54285714 0.55714286 0.57142857 0.58571429 0.6 0.61428571 0.62857143 0.64285714 0.65714286 0.67142857 0.68571429 0.7 0.71428571 0.72857143 0.74285714 0.75714286 0.77142857 0.78571429 0.8 0.81428571 0.82857143 0.84285714 0.85714286 0.87142857 0.88571429 0.9 0.91428571 0.92857143 0.94285714 0.95714286 0.97142857 0.98571429 1 1 1 1 1 1
  line L1742 (225.4942, 90.4458) -> (225.501, 90.4157) construction
  line L1743 (225.501, 90.4157) -> (225.5153, 90.3556) construction
  line L1744 (225.5153, 90.3556) -> (225.5391, 90.2662) construction
  line L1745 (225.5391, 90.2662) -> (225.5755, 90.1483) construction
  line L1746 (225.5755, 90.1483) -> (225.6271, 90.0027) construction
  line L1747 (225.6271, 90.0027) -> (225.6831, 89.8584) construction
  line L1748 (225.6831, 89.8584) -> (225.7419, 89.7148) construction
  line L1749 (225.7419, 89.7148) -> (225.8021, 89.5717) construction
  line L1750 (225.8021, 89.5717) -> (225.8633, 89.4289) construction
  line L1751 (225.8633, 89.4289) -> (225.9255, 89.2864) construction
  line L1752 (225.9255, 89.2864) -> (225.9891, 89.1443) construction
  line L1753 (225.9891, 89.1443) -> (226.0546, 89.0029) construction
  line L1754 (226.0546, 89.0029) -> (226.1222, 88.8621) construction
  line L1755 (226.1222, 88.8621) -> (226.192, 88.7221) construction
  line L1756 (226.192, 88.7221) -> (226.2636, 88.5827) construction
  line L1757 (226.2636, 88.5827) -> (226.337, 88.4439) construction
  line L1758 (226.337, 88.4439) -> (226.4117, 88.3056) construction
  line L1759 (226.4117, 88.3056) -> (226.4877, 88.1678) construction
  line L1760 (226.4877, 88.1678) -> (226.5647, 88.0303) construction
  line L1761 (226.5647, 88.0303) -> (226.6429, 87.8933) construction
  line L1762 (226.6429, 87.8933) -> (226.7224, 87.7568) construction
  line L1763 (226.7224, 87.7568) -> (226.8031, 87.6208) construction
  line L1764 (226.8031, 87.6208) -> (226.885, 87.4852) construction
  line L1765 (226.885, 87.4852) -> (226.9683, 87.3502) construction
  line L1766 (226.9683, 87.3502) -> (227.0528, 87.2157) construction
  line L1767 (227.0528, 87.2157) -> (227.1384, 87.0816) construction
  line L1768 (227.1384, 87.0816) -> (227.2252, 86.948) construction
  line L1769 (227.2252, 86.948) -> (227.313, 86.8148) construction
  line L1770 (227.313, 86.8148) -> (227.4018, 86.682) construction
  line L1771 (227.4018, 86.682) -> (227.4917, 86.5497) construction
  line L1772 (227.4917, 86.5497) -> (227.5826, 86.4179) construction
  line L1773 (227.5826, 86.4179) -> (227.6745, 86.2865) construction
  line L1774 (227.6745, 86.2865) -> (227.7674, 86.1555) construction
  line L1775 (227.7674, 86.1555) -> (227.8613, 86.025) construction
  line L1776 (227.8613, 86.025) -> (227.9562, 85.895) construction
  line L1777 (227.9562, 85.895) -> (228.052, 85.7654) construction
  line L1778 (228.052, 85.7654) -> (228.1488, 85.6362) construction
  line L1779 (228.1488, 85.6362) -> (228.2466, 85.5074) construction
  line L1780 (228.2466, 85.5074) -> (228.3452, 85.3791) construction
  line L1781 (228.3452, 85.3791) -> (228.4447, 85.2512) construction
  line L1782 (228.4447, 85.2512) -> (228.5451, 85.1238) construction
  line L1783 (228.5451, 85.1238) -> (228.6464, 84.9968) construction
  line L1784 (228.6464, 84.9968) -> (228.7486, 84.8702) construction
  line L1785 (228.7486, 84.8702) -> (228.8516, 84.744) construction
  line L1786 (228.8516, 84.744) -> (228.9555, 84.6183) construction
  line L1787 (228.9555, 84.6183) -> (229.0603, 84.493) construction
  line L1788 (229.0603, 84.493) -> (229.1658, 84.3682) construction
  line L1789 (229.1658, 84.3682) -> (229.2722, 84.2438) construction
  line L1790 (229.2722, 84.2438) -> (229.3794, 84.1198) construction
  line L1791 (229.3794, 84.1198) -> (229.4875, 83.9962) construction
  line L1792 (229.4875, 83.9962) -> (229.5963, 83.8731) construction
  line L1793 (229.5963, 83.8731) -> (229.7059, 83.7503) construction
  line L1794 (229.7059, 83.7503) -> (229.8162, 83.6281) construction
  line L1795 (229.8162, 83.6281) -> (229.9274, 83.5062) construction
  line L1796 (229.9274, 83.5062) -> (230.0393, 83.3848) construction
  line L1797 (230.0393, 83.3848) -> (230.152, 83.2638) construction
  line L1798 (230.152, 83.2638) -> (230.2655, 83.1432) construction
  line L1799 (230.2655, 83.1432) -> (230.3797, 83.0231) construction
  line L1800 (230.3797, 83.0231) -> (230.4946, 82.9034) construction
  line L1801 (230.4946, 82.9034) -> (230.6102, 82.7841) construction
  line L1802 (230.6102, 82.7841) -> (230.7266, 82.6653) construction
  line L1803 (230.7266, 82.6653) -> (230.8438, 82.5469) construction
  line L1804 (230.8438, 82.5469) -> (230.9616, 82.4289) construction
  line L1805 (230.9616, 82.4289) -> (231.0801, 82.3113) construction
  line L1806 (231.0801, 82.3113) -> (231.1994, 82.1942) construction
  line L1807 (231.1994, 82.1942) -> (231.3193, 82.0775) construction
  line L1808 (231.3193, 82.0775) -> (231.4399, 81.9612) construction
  line L1809 (231.4399, 81.9612) -> (231.5613, 81.8454) construction
  line L1810 (231.5613, 81.8454) -> (231.6832, 81.73) construction
  line L1811 (231.6832, 81.73) -> (231.8059, 81.615) construction
  line L1812 (231.8059, 81.615) -> (231.9046, 81.5233) construction
  line L1813 (231.9046, 81.5233) -> (231.9789, 81.4548) construction
  line L1814 (231.9789, 81.4548) -> (232.0286, 81.4092) construction
  line L1815 (232.0286, 81.4092) -> (232.0535, 81.3864) construction
  line L1816 (266.6686, 173.5481) -> (268.1665, 174.1948)
  arc A61 (184.5338, 99.6279) -> (181.8522, 98.8934) centre (183.5728, 97.8739) ccw
  arc A62 (264.0674, 174.5301) -> (262.5041, 177.5982) centre (212.132, 150) ccw
  line L1817 (172.8837, 105.4094) -> (171.8057, 104.1847)
  arc A63 (264.0674, 174.5301) -> (266.6686, 173.5481) centre (265.8758, 175.3842) ccw
  arc A64 (172.8837, 105.4094) -> (172.7536, 108.1868) centre (171.3824, 106.7308) ccw
  arc A65 (199.127, 207.9623) -> (201.4504, 206.435) centre (201.0785, 208.4001) ccw
  line L1818 (181.8522, 98.8934) -> (181.0205, 97.4897)
  line L1819 (181.8522, 98.8934) -> (181.0205, 97.4897)
  arc A66 (184.5338, 99.6279) -> (181.8522, 98.8934) centre (183.5728, 97.8739) ccw
  line L1820 (199.127, 207.9623) -> (198.7698, 209.5542)
  line L1821 (172.8837, 105.4094) -> (171.8057, 104.1847)
  arc A67 (172.8837, 105.4094) -> (172.7536, 108.1868) centre (171.3824, 106.7308) ccw
  line L1822 (199.127, 207.9623) -> (198.7698, 209.5542)
  spline S24 degree 5 poles (198.7698, 90.4458) (198.763, 90.4157) (198.7487, 90.3556) (198.7249, 90.2662) (198.6885, 90.1483) (198.6369, 90.0027) (198.5809, 89.8584) (198.5221, 89.7148) (198.4619, 89.5717) (198.4007, 89.4289) (198.3385, 89.2864) (198.2749, 89.1443) (198.2094, 89.0029) (198.1418, 88.8621) (198.072, 88.7221) (198.0004, 88.5827) (197.927, 88.4439) (197.8523, 88.3056) (197.7763, 88.1678) (197.6993, 88.0303) (197.6211, 87.8933) (197.5416, 87.7568) (197.4609, 87.6208) (197.379, 87.4852) (197.2957, 87.3502) (197.2112, 87.2157) (197.1256, 87.0816) (197.0388, 86.948) (196.951, 86.8148) (196.8622, 86.682) (196.7723, 86.5497) (196.6814, 86.4179) (196.5895, 86.2865) (196.4966, 86.1555) (196.4027, 86.025) (196.3078, 85.895) (196.212, 85.7654) (196.1152, 85.6362) (196.0174, 85.5074) (195.9188, 85.3791) (195.8193, 85.2512) (195.7189, 85.1238) (195.6176, 84.9968) (195.5154, 84.8702) (195.4124, 84.744) (195.3085, 84.6183) (195.2037, 84.493) (195.0982, 84.3682) (194.9918, 84.2438) (194.8846, 84.1198) (194.7765, 83.9962) (194.6677, 83.8731) (194.5581, 83.7503) (194.4478, 83.6281) (194.3366, 83.5062) (194.2247, 83.3848) (194.112, 83.2638) (193.9985, 83.1432) (193.8843, 83.0231) (193.7694, 82.9034) (193.6538, 82.7841) (193.5374, 82.6653) (193.4202, 82.5469) (193.3024, 82.4289) (193.1839, 82.3113) (193.0646, 82.1942) (192.9447, 82.0775) (192.8241, 81.9612) (192.7027, 81.8454) (192.5808, 81.73) (192.4581, 81.615) (192.3594, 81.5233) (192.2851, 81.4548) (192.2354, 81.4092) (192.2105, 81.3864) knots 0 0 0 0 0 0 0.01428571 0.02857143 0.04285714 0.05714286 0.07142857 0.08571429 0.1 0.11428571 0.12857143 0.14285714 0.15714286 0.17142857 0.18571429 0.2 0.21428571 0.22857143 0.24285714 0.25714286 0.27142857 0.28571429 0.3 0.31428571 0.32857143 0.34285714 0.35714286 0.37142857 0.38571429 0.4 0.41428571 0.42857143 0.44285714 0.45714286 0.47142857 0.48571429 0.5 0.51428571 0.52857143 0.54285714 0.55714286 0.57142857 0.58571429 0.6 0.61428571 0.62857143 0.64285714 0.65714286 0.67142857 0.68571429 0.7 0.71428571 0.72857143 0.74285714 0.75714286 0.77142857 0.78571429 0.8 0.81428571 0.82857143 0.84285714 0.85714286 0.87142857 0.88571429 0.9 0.91428571 0.92857143 0.94285714 0.95714286 0.97142857 0.98571429 1 1 1 1 1 1
  line L1823 (198.7698, 90.4458) -> (198.763, 90.4157) construction
  line L1824 (198.763, 90.4157) -> (198.7487, 90.3556) construction
  line L1825 (198.7487, 90.3556) -> (198.7249, 90.2662) construction
  line L1826 (198.7249, 90.2662) -> (198.6885, 90.1483) construction
  line L1827 (198.6885, 90.1483) -> (198.6369, 90.0027) construction
  line L1828 (198.6369, 90.0027) -> (198.5809, 89.8584) construction
  line L1829 (198.5809, 89.8584) -> (198.5221, 89.7148) construction
  line L1830 (198.5221, 89.7148) -> (198.4619, 89.5717) construction
  line L1831 (198.4619, 89.5717) -> (198.4007, 89.4289) construction
  line L1832 (198.4007, 89.4289) -> (198.3385, 89.2864) construction